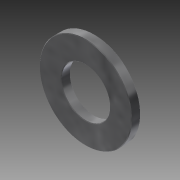
# Autodesk Inventor part: M8_Ring
Saved by Autodesk Inventor 2015 (Build 190159000, 159)
## iProperties
Created: 2015-01-09
Part Number: M8_Ring
Material: Stainless Steel
Document SubType Name: Modeling
Designer: ice
Density: 8 g/cm^3
Appearance: Semi-Polished
Mass: 1.85811 g
Surface Area: 4.04956 cm^2
Volume: 0.232264 cm^3
Author: ice
Autodesk Inventor part; units mm, degrees
ref_plane "YZ Plane" through (0, 0, 0) normal (1, 0, 0) x (0, 1, 0)
ref_plane "XZ Plane" through (0, 0, 0) normal (0, 1, 0) x (-1, 0, 0)
ref_plane "XY Plane" through (0, 0, 0) normal (0, 0, 1) x (1, 0, 0)
sketch "Sketch1" plane through (0, 0, 0) normal (0, 1, 0) x (-1, 0, 0)
  circle A0 centre (0, 0) radius 4.2
  circle A1 centre (0, 0) radius 8
  dimension "d4" = 8.4
  dimension "d5" = 16
  constraints: 2 centre point, 1 coincident
  measures "d4" diameter of A0
  measures "d5" diameter of A1
extrude "Extrusion1" add sketch "Sketch1" along normal blind 1.6
chamfer "Chamfer1" distance 0.1 angle 45 4 edges at (8, 1.6, 0) (4.2, 1.6, 0) (8, 0, 0) (4.2, 0, 0)
body "Solid1"
